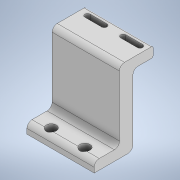
# Autodesk Inventor part: MagnetActuatorHolder
Saved by Autodesk Inventor 2021 (Build 250183000, 183)
## iProperties
Created: 2021-12-05
Part Number: MagnetActuatorHolder
Material: Generic
Document SubType Name: Modeling
Designer: Jorian Brusind
Density: 1 g/cm^3
Appearance: Default
Author: Jorian Brusind
Autodesk Inventor part; units mm, degrees
ref_plane "YZ Plane" through (0, 0, 0) normal (1, 0, 0) x (0, 1, 0)
ref_plane "XZ Plane" through (0, 0, 0) normal (0, 1, 0) x (-1, 0, 0)
ref_plane "XY Plane" through (0, 0, 0) normal (0, 0, 1) x (1, 0, 0)
sketch "Sketch1" plane through (0, 0, 0) normal (0, 1, 0) x (-1, 0, 0)
  line L0 (0, 0) -> (34, 0)
  line L1 (34, 0) -> (34, -2)
  line L2 (34, -2) -> (0, -2)
  line L3 (0, -2) -> (0, 0)
  line L4 (37, -5) -> (37, 3)
  line L5 (37, 3) -> (-3, 3)
  line L6 (-3, 3) -> (-3, -5)
  line L7 (-3, -5) -> (37, -5)
  dimension "d0" = 34
  dimension "d1" = 2
  dimension "d2" = 3
  constraints: 16 end point, 4 parallel, 2 perpendicular, 1 horizontal, 3 other
  measures "d0" distance of L1.end L2.end
  measures "d1" distance of L0.end L1.end
  measures "d2" distance between parallel lines of L1 L4
extrude "Extrusion1" add sketch "Sketch1" along normal blind 48 contours L0 L1 L2 L3 | L7 L6 L5 L4
sketch "Sketch3" plane through (0, 0, 0) normal (0, -1, 0) x (1, 0, 0)
  line L0 (-37, 3) -> (3, 3) projected
  line L1 (-37, 3) -> (3, 3)
  line L2 (3, 3) -> (3, 18)
  line L3 (3, 18) -> (-37, 18)
  line L4 (-37, 18) -> (-37, 3)
  line L5 (3, -5) -> (-37, -5) projected
  line L6 (-37, -5) -> (3, -5)
  line L7 (3, -5) -> (3, -20)
  line L8 (3, -20) -> (-37, -20)
  line L9 (-37, -20) -> (-37, -5)
  circle A0 centre (-27, -12.5) radius 3
  circle A1 centre (-27, 13.5) radius 3
  circle A2 centre (-7, -12.5) radius 3
  circle A3 centre (-7, 13.5) radius 3
  point P0 (0, 0)
  point P1 (3, -5)
  dimension "d5" = 40
  dimension "d6" = 15
  dimension "d7" = 40
  dimension "d8" = 15
  dimension "d9" = 6
  dimension "d10" = 10
  dimension "d11" = 7.5
  dimension "d14" = 26
  dimension "d17" = 20
  constraints: 16 end point, 4 centre point, 4 parallel, 3 horizontal, 2 perpendicular, 1 vertical, 6 other
  measures "d5" distance of L3.end L2.end
  measures "d6" distance of L2.end L1.end
  measures "d7" distance of L7.end L8.end
  measures "d8" distance of L6.end L7.end
  measures "d9" diameter of A0
  measures "d10" distance from line of L9 A0.centre
  measures "d11" distance from line of L8 A0.centre
  measures "d14" distance of A0.centre A1.centre
  measures "d17" distance of A0.centre A2.centre
extrude "Extrusion2" add sketch "Sketch3" against normal blind 6 contours L4 L3 L2 L0
sketch "Sketch5" plane through (0, 48, 0) normal (0, 1, 0) x (1, 0, 0)
  line L0 (3, 5) -> (-37, 5) projected
  line L1 (-37, 5) -> (3, 5)
  line L2 (3, 5) -> (3, 17)
  line L3 (3, 17) -> (-37, 17)
  line L4 (-37, 17) -> (-37, 5)
  line L5 (-32, 13) -> (-22, 13) construction
  line L6 (-32, 11.41) -> (-22, 11.41)
  line L7 (-22, 14.59) -> (-32, 14.59)
  arc A0 (-32, 14.59) -> (-32, 11.41) centre (-32, 13) ccw
  arc A1 (-22, 11.41) -> (-22, 14.59) centre (-22, 13) ccw
  line L8 (-32, 13) -> (-22, 13) construction
  line L9 (-22, 13) -> (-10.76, 13)
  line L10 (-22, 13) -> (-10.76, 13) construction
  line L11 (-10.76, 13) -> (-0.76, 13) construction
  line L12 (-10.76, 11.41) -> (-0.76, 11.41)
  line L13 (-0.76, 14.59) -> (-10.76, 14.59)
  arc A2 (-10.76, 14.59) -> (-10.76, 11.41) centre (-10.76, 13) ccw
  arc A3 (-0.76, 11.41) -> (-0.76, 14.59) centre (-0.76, 13) ccw
  point P0 (0, 0)
  point P1 (-27, 13)
  point P2 (-5.76, 13)
  point P3 (3, 5)
  dimension "d40" = 40
  dimension "d41" = 12
  dimension "d43" = 10
  dimension "d44" = 0
  dimension "d45" = 3.18
  dimension "d46" = 11.24
  dimension "d47" = 0
  dimension "d48" = 10
  dimension "d49" = 3.18
  dimension "d57" = 4
  dimension "d58" = 10
  constraints: 30 end point, 8 point on circle, 8 tangent, 6 horizontal, 4 centre point, 4 parallel, 2 collinear, 2 midpoint, 1 perpendicular
  measures "d40" distance of L3.end L2.end
  measures "d41" distance of L2.end L1.end
  measures "d43" distance of L5.start L5.end
  measures "d44" distance between parallel lines of L5 L8
  measures "d45" diameter of A1
  measures "d46" distance of L8.end L9.end
  measures "d47" distance between parallel lines of L9 L10
  measures "d48" distance of L10.end L11.end
  measures "d49" diameter of A3
  measures "d57" distance from line of L3 L5.start
  measures "d58" distance from line of L4 point (-27, 13)
extrude "Extrusion4" add sketch "Sketch5" against normal blind 6
fillet "Fillet1" radius 3 1 edges at (-17, 42, -5)
fillet "Fillet2" radius 3 2 edges at (-17, 48, 3) (-17, 6, 3)
fillet "Fillet3" radius 3 1 edges at (-17, 6, 18)
fillet "Fillet4" radius 3 1 edges at (-17, 0, -5)
fillet "Fillet5" radius 1 2 edges at (-17, 48, -17) (-17, 42, -17)
body "Solid1"
